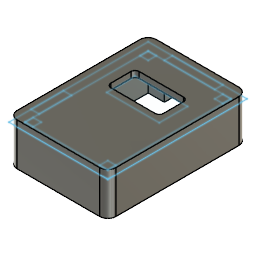
soilmeter_top (Autodesk Fusion 360 design; units mm, degrees)
part number: 2026-05-25-18-02-36-649
Autodesk Fusion 360 part; units mm, degrees
sketch "Sketch1" plane through (0, 0, 0) normal (0, 0, 1) x (1, 0, 0)
  line L0 (-15, 20) -> (26, 20)
  line L1 (26, 20) -> (26, -41)
  line L2 (26, -41) -> (-15, -41)
  line L3 (-15, -41) -> (-15, 20)
  line L4 (-7.5, 6) -> (18.5, 6)
  line L5 (18.5, 6) -> (18.5, -8)
  line L6 (18.5, -8) -> (-7.5, -8)
  line L7 (-7.5, -8) -> (-7.5, 6)
  line L8 (-19, 24) -> (30, 24)
  line L9 (30, 24) -> (30, -45)
  line L10 (30, -45) -> (-19, -45)
  line L11 (-19, -45) -> (-19, 24)
  line L12 (-15, -34) -> (-19, -34)
  line L13 (-19, -34) -> (-19, -18)
  line L14 (-19, -18) -> (-15, -18)
  line L15 (-15, -18) -> (-15, -34)
  line L16 (-15, 20) -> (-11, 20)
  line L17 (-11, 20) -> (-11, 16)
  line L18 (-11, 16) -> (-15, 16)
  line L19 (-15, 16) -> (-15, 20)
  line L20 (26, 20) -> (22, 20)
  line L21 (22, 20) -> (22, 16)
  line L22 (22, 16) -> (26, 16)
  line L23 (26, 16) -> (26, 20)
  line L24 (-15, -41) -> (-11, -41)
  line L25 (-11, -41) -> (-11, -37)
  line L26 (-11, -37) -> (-15, -37)
  line L27 (-15, -37) -> (-15, -41)
  line L28 (26, -41) -> (22, -41)
  line L29 (22, -41) -> (22, -37)
  line L30 (22, -37) -> (26, -37)
  line L31 (26, -37) -> (26, -41)
  line L32 (18, 24) -> (-7, 24)
  line L33 (-7, 24) -> (-7, 20)
  line L34 (-7, 20) -> (18, 20)
  line L35 (18, 20) -> (18, 24)
  dimension "d1" = 41
  dimension "d2" = 61
  dimension "d3" = 7.5
  dimension "d4" = 7.5
  dimension "d5" = 33
  dimension "d6" = 14
  dimension "d7" = 4
  dimension "d8" = 4
  dimension "d9" = 4
  dimension "d10" = 4
  dimension "d11" = 7
  dimension "d12" = 16
  dimension "d13" = 4
  dimension "d14" = 4
  dimension "d15" = 4
  dimension "d16" = 4
  dimension "d17" = 4
  dimension "d18" = 4
  dimension "d19" = 4
  dimension "d20" = 4
  dimension "d23" = 12
  dimension "d24" = 12
  constraint horizontal L0
  constraint vertical L1
  constraint horizontal L2
  constraint vertical L3
  constraint horizontal L4
  constraint vertical L5
  constraint horizontal L6
  constraint vertical L7
  constraint horizontal L8
  constraint vertical L9
  constraint horizontal L10
  constraint vertical L11
  constraint horizontal L12
  constraint vertical L13
  constraint horizontal L14
  constraint vertical L15
  constraint coincident L11 L13.end
  constraint coincident L3 L12.start
  constraint horizontal L16
  constraint vertical L17
  constraint horizontal L18
  constraint vertical L19
  constraint horizontal L20
  constraint vertical L21
  constraint horizontal L22
  constraint vertical L23
  constraint horizontal L24
  constraint vertical L25
  constraint horizontal L26
  constraint vertical L27
  constraint horizontal L28
  constraint vertical L29
  constraint horizontal L30
  constraint vertical L31
  constraint horizontal L32
  constraint vertical L33
  constraint horizontal L34
  constraint vertical L35
  constraint coincident L0 L33.end
  constraint coincident L8 L32.start
  measures "d1" distance of L0.start L0.end
  measures "d2" distance of L0.start L2.end
  measures "d3" distance of L3 L4.start
  measures "d4" distance of L1 L5
  measures "d5" distance of L2 L6
  measures "d6" distance of L0 L4
  measures "d7" distance of L2 L10
  measures "d8" distance of L3 L11
  measures "d9" distance of L1 L9
  measures "d10" distance of L0 L8
  measures "d11" distance of L2 L12
  measures "d12" distance of L12 L14
  measures "d13" distance of L0.start L16.end
  measures "d14" distance of L0.start L18.end
  measures "d15" distance of L0.end L20.end
  measures "d16" distance of L0.end L22.end
  measures "d17" distance of L2.end L24.end
  measures "d18" distance of L2.end L26.end
  measures "d19" distance of L1.end L28.end
  measures "d20" distance of L1.end L30.end
  measures "d23" distance of L9 L35
  measures "d24" distance of L11 L33
extrude "Extrude1" add sketch "Sketch1" along normal blind 3 makes body 1
extrude "Extrude2" add sketch "Sketch1" against normal blind 6 separate body contours L0 L3 L16 L17 L18 L19 | L0 L1 L20 L21 L22 L23 | L2 L3 L24 L25 L26 L27 | L1 L2 L28 L29 L30 L31 makes body 2 at (-13.6667, 20, -2) makes body 3 at (-12.3333, -37, -2) makes body 4 at (23.3333, 20, -2) makes body 5 at (26, -38.3333, -2)
extrude "Extrude3" add sketch "Sketch1" against normal blind 18 separate body contours L0 L3 L8 L11 L14 L16 L19 L33 | L0 L1 L2 L3 L8 L9 L10 L11 L12 L20 L23 L24 L27 L28 L31 L35 makes body 6 at (30, 1, -12) makes body 7 at (-19, -4, -6)
fillet "Fillet1" radius 2 4 edges at (-7.5, 6, 1.5) (18.5, 6, 1.5) (18.5, -8, 1.5) (-7.5, -8, 1.5) on bodies 1
fillet "Fillet2" radius 4 8 edges at (-19, -45, 1.5) (30, -45, 1.5) (30, 24, 1.5) (-19, 24, 1.5) (-19, -45, -9) (30, -45, -9) (30, 24, -9) (-19, 24, -9) on bodies 1 6 7
extrude "Extrude4" add sketch "Sketch1" against normal blind 6 contours L0 L8 L32 L33 L34 L35 bodies 1 6 7
fillet "Fillet3" radius 2 2 edges at (18, 22, -6) (-7, 22, -6) on bodies 1
fillet "Fillet4" radius 3 4 edges at (-11, 16, -3) (-11, -37, -3) (22, 16, -3) (22, -37, -3) on bodies 2 3 4 5
